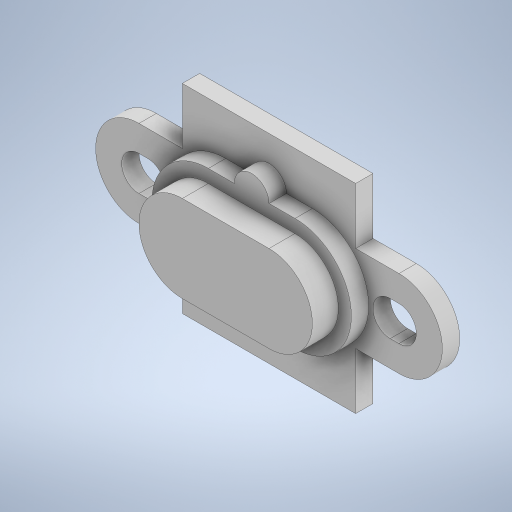
# Autodesk Inventor part: TF-LC02 (Laser senzor)
Saved by Autodesk Inventor 2024 (Build 280153000, 153)
## iProperties
Created: 2023-10-20
Part Number: TF-LC02 (Laser senzor)
Material: Všeobecné
Document SubType Name: Modeling
Designer: jaryj
Density: 1 g/cm^3
Appearance: Výchozí
Author: jaryj
Autodesk Inventor part; units mm, degrees
ref_plane "YZ Plane" through (0, 0, 0) normal (1, 0, 0) x (0, 1, 0)
ref_plane "XZ Plane" through (0, 0, 0) normal (0, 1, 0) x (-1, 0, 0)
ref_plane "XY Plane" through (0, 0, 0) normal (0, 0, 1) x (1, 0, 0)
sketch "Náčrt1" plane through (0, 0, 0) normal (0, 0, 1) x (1, 0, 0)
  line L0 (-5, 5.75) -> (5, 5.75)
  line L1 (5, -5.75) -> (-5, -5.75)
  line L2 (-5, 5.75) -> (5, -5.75) construction
  line L3 (5, 5.75) -> (-5, -5.75) construction
  line L4 (-5, 2.5) -> (-7.5, 2.5)
  arc A0 (-7.5, 2.5) -> (-7.5, -2.5) centre (-7.5, 0) ccw
  line L5 (-7.5, -2.5) -> (-5, -2.5)
  line L6 (5, 2.5) -> (7.5, 2.5)
  arc A1 (7.5, -2.5) -> (7.5, 2.5) centre (7.5, 0) ccw
  line L7 (7.5, -2.5) -> (5, -2.5)
  line L8 (-5, -5.75) -> (-5, -2.5)
  line L9 (-5, 2.5) -> (-5, 5.75)
  line L10 (5, 5.75) -> (5, 2.5)
  line L11 (5, -2.5) -> (5, -5.75)
  line L12 (-7.5, 0) -> (-7, 0) construction
  line L13 (-7.5, -1) -> (-7, -1)
  line L14 (-7, 1) -> (-7.5, 1)
  arc A2 (-7.5, 1) -> (-7.5, -1) centre (-7.5, 0) ccw
  arc A3 (-7, -1) -> (-7, 1) centre (-7, 0) ccw
  line L15 (7.5, 0) -> (7, 0) construction
  line L16 (7.5, 1) -> (7, 1)
  line L17 (7, -1) -> (7.5, -1)
  arc A4 (7.5, -1) -> (7.5, 1) centre (7.5, 0) ccw
  arc A5 (7, 1) -> (7, -1) centre (7, 0) ccw
  point P0 (0, 0)
  point P1 (-7.25, 0)
  point P2 (7.25, 0)
  point P3 (10, 0)
  point P4 (-10, 0)
  point P5 (-6, 0)
  point P6 (-8.5, 0)
  dimension "d0" = 11.5
  dimension "d1" = 10
  dimension "d2" = 5
  dimension "d3" = 2
  dimension "d4" = 20
  dimension "d5" = 2.5
  constraints: 40 end point, 16 point on circle, 12 tangent, 7 parallel, 6 centre point, 6 perpendicular, 4 horizontal, 4 horizontal alignment, 4 midpoint, 2 collinear, 1 point on line, 1 vertical alignment
  measures "d0" distance between parallel lines of L1 L0
  measures "d1" distance between parallel lines of L10 L9
  measures "d2" distance between parallel lines of L5 L4
  measures "d3" distance between parallel lines of L17 L16
  measures "d4" distance of point (10, 0) point (-10, 0)
  measures "d5" distance of point (-6, 0) point (-8.5, 0)
extrude "Vysunutí1" add sketch "Náčrt1" along normal blind 1
sketch "Náčrt2" plane through (0, 0, 1) normal (0, 0, 1) x (1, 0, 0)
  line L0 (-2.5, 0) -> (2.5, 0) construction
  line L1 (2.5, -3.25) -> (-2.5, -3.25)
  arc A0 (-2.5, 3.25) -> (-2.5, -3.25) centre (-2.5, 0) ccw
  arc A1 (2.5, -3.25) -> (2.5, 3.25) centre (2.5, 0) ccw
  arc A2 (1, 3.25) -> (-1, 3.25) centre (0, 3.25) ccw
  line L2 (-2.5, 3.25) -> (-1, 3.25)
  line L3 (1, 3.25) -> (2.5, 3.25)
  point P0 (0, 0)
  point P1 (5.75, 0)
  point P2 (-5.75, 0)
  dimension "d8" = 6.5
  dimension "d9" = 11.5
  dimension "d10" = 1
  constraints: 10 end point, 8 point on circle, 6 tangent, 3 centre point, 2 parallel, 1 horizontal, 1 horizontal alignment, 1 midpoint, 1 vertical alignment
  measures "d8" distance between parallel lines of L1 L3
  measures "d9" distance of point (5.75, 0) point (-5.75, 0)
  measures "d10" radius of A2
extrude "Vysunutí2" add sketch "Náčrt2" along normal blind 1
sketch "Náčrt3" plane through (0, 0, 2) normal (0, 0, 1) x (1, 0, 0)
  arc A0 (-2.5, 3.25) -> (-2.5, -3.25) centre (-2.5, 0) ccw projected
  line L0 (-1, 3.25) -> (-2.5, 3.25) projected
  line L1 (2.5, 3.25) -> (1, 3.25) projected
  arc A1 (2.5, -3.25) -> (2.5, 3.25) centre (2.5, 0) ccw projected
  line L2 (-2.5, -3.25) -> (2.5, -3.25) projected
  line L3 (-1, 3.25) -> (1, 3.25)
  line L4 (2.5, 2.5) -> (1, 2.5)
  line L5 (1, 2.5) -> (-1, 2.5)
  line L6 (-1, 2.5) -> (-2.5, 2.5)
  arc A2 (-2.5, 2.5) -> (-2.5, -2.5) centre (-2.5, 0) ccw
  line L7 (-2.5, -2.5) -> (2.5, -2.5)
  arc A3 (2.5, -2.5) -> (2.5, 2.5) centre (2.5, 0) ccw
  point P0 (0, 0)
  dimension "d13" = 0.75
  constraints: 10 end point, 4 point on circle, 2 centre point, 1 horizontal, 5 other
  measures "d13" radial gap between concentric circles of A1 A3
extrude "Vysunutí3" add sketch "Náčrt3" along normal blind 1.5 contours A3 L7 A2 L6 L5 L4
